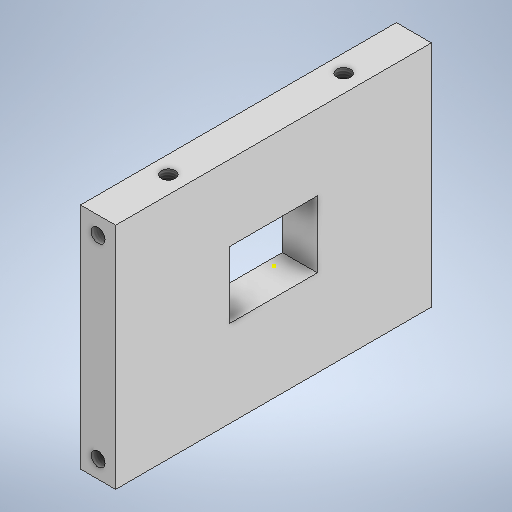
# Autodesk Inventor part: Rb PEEK - Largo
Saved by Autodesk Inventor 2025.3 (Build 293356000, 356)
## iProperties
Created: 2025-05-09
Part Number: Rb PEEK - Largo
Material: Generic
Document SubType Name: Modeling
Designer: E. Moreno
Density: 1 g/cm^3
Appearance: Default
Categories: <MemberInstance><Categories><Category DisplayName="" Mnemonic="CABLEANDHARNESS" InternalName="e4a7e005-5e42-4d16-b293-125e7f0d0512"><Category DisplayName="" Mnemonic="CONNECTORS" InternalName="6f634eba-a678-4820-a31d-2c2d5ee6728e"><CategoryParameter DisplayName="" Mnemonic="REFDES" InternalName="c3740e8c-60ab-4d5d-8584-52b73222f2f0"/><Category DisplayName="" Mnemonic="DISCRETEWIRE" InternalName="9a3407de-09b2-4cdb-8c40-9708d5144a28"/></Category></Category></Categories><FamilyTemplate><FamilyTemplateParameters></FamilyTemplateParameters></FamilyTemplate><CategoryParameterMap><ParamToTemplateMap><ParamToTemplate CategoryParameter="//CategoryParameter[@InternalName='c3740e8c-60ab-4d5d-8584-52b73222f2f0']" ConstantValue=""/></ParamToTemplateMap></CategoryParameterMap></MemberInstance>
Author: E. Moreno
Title: Rb PEEK - Largo
Autodesk Inventor part; units mm, degrees
ref_plane "YZ Plane" through (0, 0, 0) normal (1, 0, 0) x (0, 1, 0)
ref_plane "XZ Plane" through (0, 0, 0) normal (0, 1, 0) x (-1, 0, 0)
ref_plane "XY Plane" through (0, 0, 0) normal (0, 0, 1) x (1, 0, 0)
sketch "Sketch1" plane through (0, 0, 0) normal (1, 0, 0) x (0, 1, 0)
  line L0 (-32.6, 45) -> (32.6, 45)
  line L1 (32.6, 45) -> (32.6, -45)
  line L2 (32.6, -45) -> (-32.6, -45)
  line L3 (-32.6, -45) -> (-32.6, 45)
  line L4 (-32.6, 45) -> (32.6, -45) construction
  line L5 (32.6, 45) -> (-32.6, -45) construction
  point P0 (0, 0)
  dimension "d0" = 65.2
  dimension "d1" = 90
  constraints: 12 end point, 2 midpoint, 2 parallel, 1 horizontal, 1 perpendicular
  measures "d0" distance of L1.end L2.end
  measures "d1" distance of L0.end L1.end
extrude "Extrusion1" add sketch "Sketch1" along normal blind 10
sketch "Sketch2" plane through (0, 32.6, 45) normal (0, 1, 0) x (1, 0, 0)
  line L0 (0, 0) -> (10, 0) projected
  line L1 (0, 0) -> (5, 0)
  line L2 (5, 0) -> (5, 20)
  circle A0 centre (5, 20) radius 2
  line L3 (0, 45) -> (10, 45)
  line L4 (0, 90) -> (10, 90)
  line L5 (0, 90) -> (5, 90)
  line L6 (5, 90) -> (5, 70)
  circle A1 centre (5, 70) radius 2
  dimension "d4" = 5
  dimension "d5" = 20
  dimension "d6" = 4
  constraints: 12 end point, 5 symmetric about line, 2 centre point, 2 coincident, 1 horizontal, 1 midpoint, 1 perpendicular, 1 other
  measures "d4" distance of L0.start L1.end
  measures "d5" distance of L1.end L2.end
  measures "d6" diameter of A0
extrude "Extrusion2" cut sketch "Sketch2" against normal blind 25
thread "Thread1" size "M4x0.7" class "6H" standard "ANSI Metric M Profile" full length
thread "Thread2" size "M4x0.7" class "6H" standard "ANSI Metric M Profile" full length
sketch "Sketch3" plane through (0, -32.6, -45) normal (0, -1, 0) x (1, 0, 0)
  line L0 (0, 45) -> (9.9068, 45)
  line L1 (10, 0) -> (10, 90) projected
  line L2 (10, 90) -> (5, 90)
  line L3 (0, 90) -> (10, 90) projected
  line L4 (5, 90) -> (5, 70)
  circle A0 centre (5, 70) radius 2
  line L5 (10, 0) -> (5, 0)
  line L6 (0, 0) -> (10, 0)
  line L7 (5, 0) -> (5, 20)
  circle A1 centre (5, 20) radius 2
  dimension "d13" = 5
  dimension "d14" = 20
  dimension "d15" = 4
  constraints: 12 end point, 4 symmetric about line, 2 centre point, 2 coincident, 1 horizontal, 1 midpoint, 1 perpendicular, 1 other
  measures "d13" distance of L1.end L2.end
  measures "d14" distance of L2.end L4.end
  measures "d15" diameter of A0
extrude "Extrusion3" cut sketch "Sketch3" against normal blind 25
thread "Thread3" size "M4x0.7" class "6H" standard "ANSI Metric M Profile" full length
thread "Thread4" size "M4x0.7" class "6H" standard "ANSI Metric M Profile" full length
sketch "Sketch6" plane through (10, 0, 0) normal (1, 0, 0) x (0, 0, -1)
  line L0 (-45, -32.6) -> (45, -32.6) projected
  line L1 (0, -32.6) -> (0, 1.6)
  line L2 (-12.5, -7.9) -> (12.5, -7.9)
  line L3 (12.5, -7.9) -> (12.5, 11.1)
  line L4 (12.5, 11.1) -> (-12.5, 11.1)
  line L5 (-12.5, 11.1) -> (-12.5, -7.9)
  line L6 (-12.5, -7.9) -> (12.5, 11.1) construction
  line L7 (12.5, -7.9) -> (-12.5, 11.1) construction
  point P0 (0, 0)
  dimension "d29" = 34.2
  dimension "d30" = 25
  dimension "d31" = 19
  constraints: 14 end point, 3 midpoint, 2 parallel, 1 horizontal, 1 perpendicular, 1 vertical
  measures "d29" distance of L1.start L1.end
  measures "d30" distance of L4.end L3.end
  measures "d31" distance of L3.end L2.end
extrude "Extrusion6" cut sketch "Sketch6" against normal blind 10
sketch "Sketch10" plane through (10, 0, 0) normal (1, 0, 0) x (0, 0, -1)
  circle A0 centre (-27.5, 25.1) radius 2.5 projected
sketch "Sketch11" plane through (0, 0, 0) normal (-1, 0, 0) x (0, 0, 1)
  circle A0 centre (27.5, 25.1) radius 2.5 projected
sketch "Sketch12" plane through (0, -32.6, 45) normal (0, 0, 1) x (1, 0, 0)
  line L0 (0, 65.2173) -> (5, 65.2173)
  line L1 (5, 65.2173) -> (5, 60.2173)
  line L2 (0, 32.6) -> (10, 32.6)
  line L3 (10, 0) -> (10, 65.2) projected
  circle A0 centre (5, 60.2173) radius 2
  circle A1 centre (5, 4.9827) radius 2
  dimension "d46" = 5
  dimension "d47" = 5
  dimension "d48" = 4
  constraints: 6 end point, 2 centre point, 2 coincident, 2 symmetric about line, 1 horizontal, 1 midpoint, 1 perpendicular, 1 other
  measures "d46" distance of L0.start L0.end
  measures "d47" distance of L0.end L1.end
  measures "d48" diameter of A0
extrude "Extrusion9" cut sketch "Sketch12" against normal blind 15
sketch "Sketch13" plane through (10, 0, 0) normal (1, 0, 0) x (0, 0, -1)
  point P0 (0, 0)
sketch "Sketch14" plane through (0, -32.6, -45) normal (0, 0, -1) x (-1, 0, 0)
  line L0 (0, 65.2) -> (-10, 65.2) projected
  line L1 (-10, 65.2) -> (-5, 65.2)
  line L2 (-5, 65.2) -> (-5, 60.2)
  circle A0 centre (-5, 60.2) radius 2
  line L3 (0, 32.6) -> (-10, 32.6)
  line L4 (-10, 43.7) -> (-10, 24.7) projected
  circle A1 centre (-5, 5) radius 2
  dimension "d51" = 5
  dimension "d52" = 5
  dimension "d53" = 4
  constraints: 6 end point, 2 centre point, 2 coincident, 2 symmetric about line, 1 horizontal, 1 midpoint, 1 perpendicular, 1 point on line, 1 other
  measures "d51" distance of L0.end L1.end
  measures "d52" distance of L1.end L2.end
  measures "d53" diameter of A0
extrude "Extrusion10" cut sketch "Sketch14" against normal blind 15
thread "Thread5" size "M4x0.7" class "6H" standard "ANSI Metric M Profile" full length
thread "Thread6" size "M4x0.7" class "6H" standard "ANSI Metric M Profile" full length
thread "Thread7" size "M4x0.7" class "6H" standard "ANSI Metric M Profile" full length
thread "Thread8" size "M4x0.7" class "6H" standard "ANSI Metric M Profile" full length
body "Solid1"
